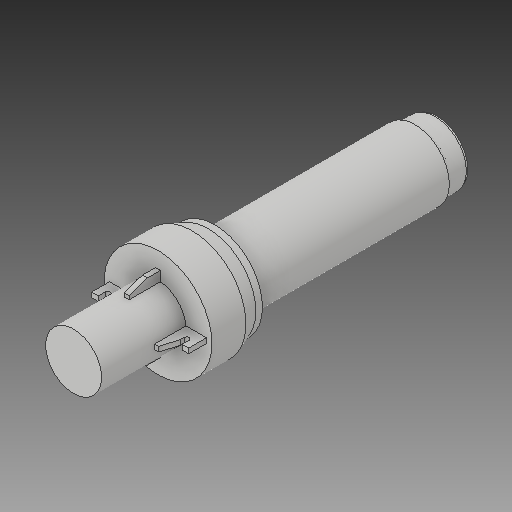
# Autodesk Inventor part: soprador_original
Saved by Autodesk Inventor 2018 (Build 220112000, 112)
## iProperties
Created: 2018-05-02
Part Number: soprador_original
Material: Genérico
Document SubType Name: Modeling
Designer: Georgines
Density: 1 g/cm^3
Appearance: Padrão
Mass: 142.66 g
Surface Area: 483.744 cm^2
Volume: 142.66 cm^3
Author: Georgines
Autodesk Inventor part; units mm, degrees
ref_plane "YZ Plane" through (0, 0, 0) normal (1, 0, 0) x (0, 1, 0)
ref_plane "XZ Plane" through (0, 0, 0) normal (0, 1, 0) x (-1, 0, 0)
ref_plane "XY Plane" through (0, 0, 0) normal (0, 0, 1) x (1, 0, 0)
sketch "Esboço2" plane through (0, 0, 0) normal (0, 0, 1) x (1, 0, 0)
  circle A0 centre (0, 0) radius 8.1
  circle A1 centre (0, 0) radius 13.9
  circle A2 centre (0, 0) radius 17.58
  line L0 (1.08, 8.0277) -> (1.08, 13.858)
  line L1 (-1.08, 13.858) -> (-1.08, 8.0277)
  line L2 (-6.4122, 4.9491) -> (-11.4614, 7.8643)
  line L3 (-12.5414, 5.9937) -> (-7.4922, 3.0785)
  line L4 (11.4614, 7.8643) -> (6.4122, 4.9491)
  line L5 (7.4922, 3.0785) -> (12.5414, 5.9937)
  line L6 (12.5414, -5.9937) -> (7.4922, -3.0785)
  line L7 (6.4122, -4.9491) -> (11.4614, -7.8643)
  line L8 (1.08, -13.858) -> (1.08, -8.0277)
  line L9 (-1.08, -8.0277) -> (-1.08, -13.858)
  line L10 (-11.4614, -7.8643) -> (-6.4122, -4.9491)
  line L11 (-7.4922, -3.0785) -> (-12.5414, -5.9937)
  dimension "d2" = 16.2
  dimension "d3" = 27.8
  dimension "d4" = 35.16
  constraints: 24 end point, 3 coincident, 1 centre point, 1 parallel, 28 other
  measures "d4" diameter of A2
extrude "Extrusão1" add sketch "Esboço2" along normal blind 0.8 contours A0 | A0 L4 A1 L5 | L6 A1 L7 A0 | A0 L1 A1 L0 | L8 A1 L9 A0 | A0 L3 A1 L2 | L10 A1 L11 A0 | A2
sketch "Esboço3" plane through (0, 0, 0.8) normal (0, 0, 1) x (1, 0, 0)
  circle A0 centre (0, 0) radius 17.58
  circle A1 centre (0, 0) radius 17.18
  dimension "d11" = 34.36
  constraints: 2 centre point, 2 coincident
  measures "d11" diameter of A1
extrude "Extrusão2" add sketch "Esboço3" along normal blind 10.3
ref_plane "Plano de trabalho3" through (0, 0, 11.1) normal (0, 0, 1) x (1, 0, 0)
sketch "Esboço4" plane through (0, 0, 11.1) normal (0, 0, 1) x (1, 0, 0)
  circle A0 centre (0, 0) radius 17.18
  circle A1 centre (0, 0) radius 19.19
  dimension "d15" = 38.38
  constraints: 2 centre point, 2 coincident
  measures "d15" diameter of A1
extrude "Extrusão3" add sketch "Esboço4" along normal blind 113.4
fillet "Arredondamento1" radius 2 1 edges at (-17.58, 0, 0)
fillet "Arredondamento2" radius 2 1 edges at (-19.19, 0, 11.1)
sketch "Esboço5" plane through (0, 0, 124.5) normal (0, 0, 1) x (1, 0, 0)
  circle A0 centre (0, 0) radius 17.18
  circle A1 centre (0, 0) radius 26.5
  circle A2 centre (-23, 0.0258) radius 1.5
  circle A3 centre (11.4777, -19.9315) radius 1.5
  circle A4 centre (11.5223, 19.9057) radius 1.5
  dimension "d21" = 53
  dimension "d23" = 3
  constraints: 5 centre point, 2 coincident
  measures "d21" diameter of A1
  measures "d23" diameter of A2
extrude "Extrusão4" add sketch "Esboço5" along normal blind 0.8
fillet "Arredondamento3" radius 2 1 edges at (-19.19, 0, 124.5)
sketch "Esboço6" plane through (0, 0, 125.3) normal (0, 0, 1) x (1, 0, 0)
  circle A0 centre (0, 0) radius 26.5
  circle A1 centre (0, 0) radius 17.18
  circle A2 centre (-23, 0.0258) radius 1.5 projected
  circle A3 centre (-23, 0.0258) radius 1.5
  circle A4 centre (11.4777, -19.9315) radius 1.5 projected
  circle A5 centre (11.4777, -19.9315) radius 1.5
  circle A6 centre (11.5223, 19.9057) radius 1.5 projected
  circle A7 centre (11.5223, 19.9057) radius 1.5
  constraints: 5 centre point, 5 coincident
extrude "Extrusão5" add sketch "Esboço6" along normal blind 2.8
sketch "Esboço9" plane through (0, 0, 128.1) normal (0, 0, 1) x (1, 0, 0)
  point P0 (0, 0)
sketch "Esboço10" plane through (0, 0, 128.1) normal (0, 0, 1) x (1, 0, 0)
  arc A0 (7.4922, -3.0785) -> (7.4922, 3.0785) centre (0, 0) ccw projected
  circle A1 centre (0, 0) radius 26.5
  constraints: 1 centre point, 1 coincident
extrude "Extrusão8" add sketch "Esboço10" along normal blind 0.1
ref_plane "Plano de trabalho7" through (0, 0, 137.2) normal (0, 0, 1) x (1, 0, 0)
sketch "Esboço11" plane through (0, 0, 137.2) normal (0, 0, 1) x (1, 0, 0)
  arc A0 (-6.4122, -4.9491) -> (-1.08, -8.0277) centre (0, 0) ccw projected
  circle A1 centre (0, 0) radius 30
  dimension "d42" = 60
  constraints: 1 centre point, 1 coincident
  measures "d42" diameter of A1
extrude "Extrusão9" add sketch "Esboço11" along normal blind 16
loft "Transição1" add section 1 edges at (-26.5, 0, 128.2) section 2 edges at (-30, 0, 137.2)
sketch "Esboço12" plane through (0, 0, 153.2) normal (0, 0, 1) x (1, 0, 0)
  circle A0 centre (0, 0) radius 15.58 projected
  circle A1 centre (0, 0) radius 30
  circle A2 centre (0, 0) radius 15
  dimension "d49" = 30
  constraints: 2 centre point, 2 coincident
  measures "d49" diameter of A2
extrude "Extrusão10" add sketch "Esboço12" along normal blind 3 contours A1
sketch "Esboço14" plane through (0, 0, 156.2) normal (0, 0, 1) x (1, 0, 0)
  circle A0 centre (0, 0) radius 15.58
  constraints: 1 centre point, 1 coincident
extrude "Extrusão11" add sketch "Esboço14" along normal blind 47
sketch "Esboço15" plane through (0, 0, 0) normal (0, 1, 0) x (-1, 0, 0)
  line L0 (15.58, 156.2) -> (15.58, 173.63)
  line L1 (15.58, 173.63) -> (17.92, 173.63)
  line L2 (15.58, 156.2) -> (27.03, 156.2)
  line L3 (30, 156.2) -> (-30, 156.2) projected
  line L4 (27.03, 156.2) -> (27.03, 166.13)
  line L5 (27.03, 166.13) -> (23.31, 166.13)
  line L6 (23.31, 166.13) -> (23.31, 162.2)
  line L7 (20.66, 162.2) -> (20.66, 164.14)
  line L8 (20.66, 164.14) -> (17.92, 173.63)
  arc A0 (20.66, 162.2) -> (23.31, 162.2) centre (21.985, 162.2) ccw
  point P0 (0, 0)
  dimension "d54" = 17.43
  dimension "d55" = 2.34
  dimension "d56" = 11.45
  dimension "d57" = 9.93
  dimension "d58" = 3.72
  dimension "d62" = 9.49
  dimension "d66" = 3.72
  dimension "d83" = 6
  dimension "d84" = 1.325
  constraints: 16 end point, 3 perpendicular, 2 point on circle, 2 tangent, 1 centre point, 1 parallel, 1 point on line
  measures "d54" distance of L0.start L0.end
  measures "d55" distance of L0.end L1.end
  measures "d56" distance of L2.start L2.end
  measures "d57" distance of L2.end L4.end
  measures "d58" distance of L4.end L5.end
  measures "d62" vertical distance of L7.end L1.end
  measures "d66" distance between parallel lines of L4 L6
  measures "d83" distance from line of L2 A0.centre
  measures "d84" radius of A0
extrude "Extrusão12" add sketch "Esboço15" along normal mid plane 2.74
pattern_circular "Padrão circular1" count 2 over 360 about axis through (0, 0, 156.2) along (0, 0, 1) of "Extrusão12"
sketch "Esboço17" plane through (0, 0, 0) normal (1, 0, 0) x (0, 1, 0)
  line L0 (15.58, 173.63) -> (17.58, 173.63)
  line L1 (15.58, 173.63) -> (15.58, 156.2)
  line L2 (15.58, 156.2) -> (15.58, 203.2) projected
  line L3 (15.58, 156.2) -> (21.03, 156.2)
  line L4 (30, 156.2) -> (-30, 156.2) projected
  line L5 (21.03, 156.2) -> (21.03, 163.48)
  line L6 (21.03, 163.48) -> (17.58, 173.63)
  point P0 (0, 0)
  dimension "d70" = 2
  dimension "d71" = 5.45
  dimension "d72" = 7.28
  constraints: 10 end point, 2 point on line, 1 horizontal, 1 vertical
  measures "d70" distance of L0.start L0.end
  measures "d71" distance of L1.end L3.end
  measures "d72" distance of L3.end L5.end
extrude "Extrusão13" add sketch "Esboço17" along normal mid plane 2.74
pattern_circular "Padrão circular2" count 2 over 360 about axis through (0, 0, 2) along (0, 0, -1) of "Extrusão13"
